Opensprinkler Shield (Autodesk Fusion 360 design; units mm, degrees)
Autodesk Fusion 360 part; units mm, degrees
sketch "Sketch1" plane through (0, 0, 0) normal (0, 0, 1) x (1, 0, 0)
  line L0 (0, 0) -> (16, 0)
  line L1 (16, 0) -> (16, 140)
  line L2 (16, 140) -> (0, 140)
  line L3 (0, 140) -> (0, 0)
  circle A0 centre (7, 128) radius 2
  circle A1 centre (7, 92) radius 2
  circle A2 centre (10, 57) radius 2
  circle A3 centre (10, 10) radius 2
  dimension "d1" = 16
  dimension "d2" = 140
  dimension "d3" = 4
  dimension "d4" = 12
  dimension "d5" = 7
  dimension "d6" = 4
  dimension "d7" = 48
  dimension "d9" = 7
  dimension "d10" = 4
  dimension "d11" = 83
  dimension "d12" = 10
  dimension "d13" = 4
  dimension "d14" = 130
  dimension "d15" = 10
  constraint horizontal L0
  constraint vertical L1
  constraint horizontal L2
  constraint vertical L3
  constraint coincident L0.start L3.end
  measures "d1" distance of L0.start L0.end
  measures "d2" distance of L0.start L2.end
  measures "d3" diameter of A0
  measures "d4" distance of L2 A0.centre
  measures "d5" distance of L3 A0.centre
  measures "d6" diameter of A1
  measures "d7" distance of L2 A1.centre
  measures "d9" distance of L3 A1.centre
  measures "d10" diameter of A2
  measures "d11" distance of L2 A2.centre
  measures "d12" distance of L3 A2.centre
  measures "d13" diameter of A3
  measures "d14" distance of L2 A3.centre
  measures "d15" distance of L3 A3.centre
extrude "Extrude1" add sketch "Sketch1" along normal blind 2.6
